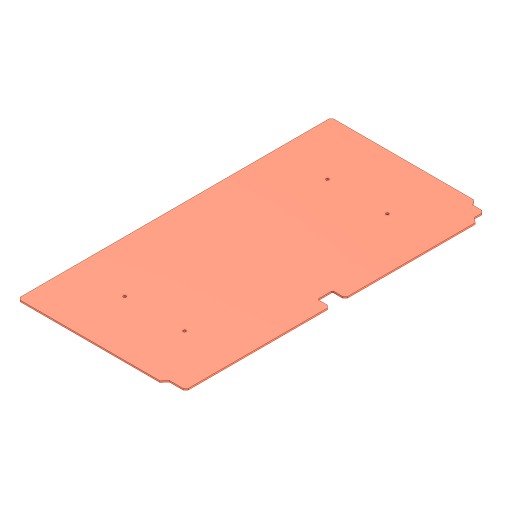
# Autodesk Inventor part: enc-BackPanel Top V2
Saved by Autodesk Inventor 2023.2 (Build 272271000, 271)
## iProperties
Created: 2023-12-04
Part Number: enc-BackPanel Top V2
Material: Generisch
Document SubType Name: Modeling
Designer: Nils Bade
Density: 1 g/cm^3
Appearance: PVC Verglasung
Description: Fertigung
Auf Bestellliste: True
Author: Nils Bade
Autodesk Inventor part; units mm, degrees
ref_plane "YZ Plane" through (0, 0, 0) normal (1, 0, 0) x (0, 1, 0)
ref_plane "XZ Plane" through (0, 0, 0) normal (0, 1, 0) x (-1, 0, 0)
ref_plane "XY Plane" through (0, 0, 0) normal (0, 0, 1) x (1, 0, 0)
sketch "Skizze1" plane through (0, 0, 0) normal (0, 1, 0) x (-1, 0, 0)
  line L0 (163.25, 314) -> (-163.25, 314)
  line L1 (-163.25, 314) -> (-163.25, -314)
  line L2 (-163.25, -314) -> (163.25, -314)
  line L3 (163.25, -314) -> (163.25, 314)
  line L4 (163.25, 314) -> (-163.25, -314) construction
  line L5 (-163.25, 314) -> (163.25, -314) construction
  line L6 (-228.55, 0) -> (228.55, 0) construction
  line L7 (0, -439.6) -> (0, 439.6) construction
  circle A0 centre (60, -203) radius 2.75
  circle A1 centre (-60, -203) radius 2.75
  circle A2 centre (60, 203) radius 2.75
  circle A3 centre (-60, 203) radius 2.75
  line L8 (-121.75, -314) -> (-130.141, -304)
  line L9 (-130.141, -304) -> (-163.25, -304)
  line L10 (-121.75, 314) -> (-130.141, 304)
  line L11 (-130.141, 304) -> (-163.25, 304)
  line L12 (-163.25, -314) -> (-153.25, -314)
  line L13 (-153.25, -314) -> (-153.25, -284)
  line L14 (-153.25, -284) -> (-163.25, -284)
  line L15 (-163.25, -284) -> (-163.25, -314)
  line L16 (-153.25, -284) -> (-163.25, -275.609)
  line L17 (-163.25, 15) -> (-138.25, 15)
  line L18 (-138.25, 15) -> (-138.25, -15)
  line L19 (-138.25, -15) -> (-163.25, -15)
  line L20 (-163.25, -15) -> (-163.25, 15)
  point P0 (0, 0)
  point P1 (-163.25, 304)
  point P2 (-153.25, -304)
  point P3 (-138.25, 0)
  dimension "d0" = 628
  dimension "d1" = 326.5
  dimension "d2" = 5.5
  dimension "d3" = 60
  dimension "d4" = 111
  dimension "d10" = 41.5
  dimension "d11" = 10
  dimension "d12" = 50
  dimension "d13" = 10
  dimension "d14" = 30
  dimension "d15" = 50
  dimension "d16" = 25
  dimension "d17" = 30
  constraints: 38 end point, 6 parallel, 6 symmetric about line, 5 point on line, 4 centre point, 4 perpendicular, 3 horizontal, 3 midpoint, 3 other
  measures "d0" distance of L2.end L0.start
  measures "d1" distance of L1.end L2.end
  measures "d2" diameter of A0
  measures "d3" distance from line of L7 A0.centre
  measures "d4" distance from line of L2 A0.centre
  measures "d10" distance from line of L1 L8.start
  measures "d11" distance between parallel lines of L2 L9
  measures "d12" angle of L2 L8
  measures "d13" distance between parallel lines of L13 L1
  measures "d14" distance between parallel lines of L12 L14
  measures "d15" angle of L1 L16
  measures "d16" distance between parallel lines of L20 L18
  measures "d17" distance between parallel lines of L17 L19
extrude "Extrusion1" add sketch "Skizze1" along normal blind 3 contours L3 L2 L8 L9 L13 L16 L1 L19 L18 L17 L11 L10 L0
chamfer "Fase-5mm" distance 5 angle 45 6 edges at (-163.25, 1.5, 314) (-163.25, 1.5, -314) (153.25, 1.5, -304) (163.25, 1.5, -15) (163.25, 1.5, 15) (163.25, 1.5, 304)
chamfer "Fase-2mm" distance 2 angle 45 2 edges at (138.25, 1.5, -15) (138.25, 1.5, 15)
